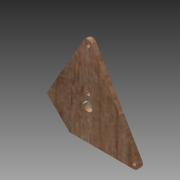
# Autodesk Inventor part: endPlateNew
Saved by Autodesk Inventor 2015 (Build 190159000, 159)
## iProperties
Created: 2014-11-20
Part Number: endPlateNew
Material: Wood (Birch)
Document SubType Name: Modeling
Designer: rawrdong
Density: 0.55 g/cm^3
Appearance: Birch - Natural Polished
Author: rawrdong
Autodesk Inventor part; units mm, degrees
ref_plane "YZ Plane" through (0, 0, 0) normal (1, 0, 0) x (0, 1, 0)
ref_plane "XZ Plane" through (0, 0, 0) normal (0, 1, 0) x (-1, 0, 0)
ref_plane "XY Plane" through (0, 0, 0) normal (0, 0, 1) x (1, 0, 0)
sketch "Sketch1" plane through (0, 0, 0) normal (0, 0, 1) x (1, 0, 0)
  arc A0 (24.3433, 15.7866) -> (20.9282, 16.7017) centre (22.1782, 14.5366) ccw projected
  line L0 (24.3433, 15.7866) -> (25.8433, 13.1886) projected
  arc A1 (24.9282, 9.7735) -> (25.8433, 13.1886) centre (23.6782, 11.9386) ccw projected
  line L1 (22.7631, 8.5235) -> (24.9282, 9.7735) projected
  arc A2 (22.7631, 8.5235) -> (22.0311, 5.7915) centre (23.7631, 6.7915) ccw projected
  line L2 (22.0311, 5.7915) -> (35.0311, -16.7252) projected
  arc A3 (32, -21.9752) -> (35.0311, -16.7252) centre (32, -18.4752) ccw projected
  line L3 (32, -21.9752) -> (6, -21.9752) projected
  arc A4 (6, -21.9752) -> (4, -23.9752) centre (6, -23.9752) ccw projected
  line L4 (4, -26.4752) -> (4, -23.9752) projected
  arc A5 (1.5, -28.9752) -> (4, -26.4752) centre (1.5, -26.4752) ccw projected
  line L5 (1.5, -28.9752) -> (-1.5, -28.9752) projected
  arc A6 (-4, -26.4752) -> (-1.5, -28.9752) centre (-1.5, -26.4752) ccw projected
  line L6 (-4, -23.9752) -> (-4, -26.4752) projected
  arc A7 (-4, -23.9752) -> (-6, -21.9752) centre (-6, -23.9752) ccw projected
  line L7 (-6, -21.9752) -> (-32, -21.9752) projected
  arc A8 (-35.0311, -16.7252) -> (-32, -21.9752) centre (-32, -18.4752) ccw projected
  line L8 (-35.0311, -16.7252) -> (-22.0311, 5.7915) projected
  arc A9 (-22.0311, 5.7915) -> (-22.7631, 8.5235) centre (-23.7631, 6.7915) ccw projected
  line L9 (-24.9282, 9.7735) -> (-22.7631, 8.5235) projected
  arc A10 (-25.8433, 13.1886) -> (-24.9282, 9.7735) centre (-23.6782, 11.9386) ccw projected
  line L10 (-25.8433, 13.1886) -> (-24.3433, 15.7866) projected
  arc A11 (-20.9282, 16.7017) -> (-24.3433, 15.7866) centre (-22.1782, 14.5366) ccw projected
  line L11 (-18.7631, 15.4517) -> (-20.9282, 16.7017) projected
  arc A12 (-18.7631, 15.4517) -> (-16.0311, 16.1838) centre (-17.7631, 17.1838) ccw projected
  line L12 (-16.0311, 16.1838) -> (-3.0311, 38.7004) projected
  arc A13 (3.0311, 38.7004) -> (-3.0311, 38.7004) centre (0, 36.9504) ccw projected
  line L13 (3.0311, 38.7004) -> (16.0311, 16.1838) projected
  arc A14 (16.0311, 16.1838) -> (18.7631, 15.4517) centre (17.7631, 17.1838) ccw projected
  line L14 (20.9282, 16.7017) -> (18.7631, 15.4517) projected
  circle A15 centre (22.6033, 13.05) radius 1.25 projected
  circle A16 centre (-22.6033, 13.05) radius 1.25 projected
  circle A17 centre (0, -26.1) radius 1.25 projected
  arc A18 (30.8494, -15.1698) -> (28.5621, -19.1315) centre (32, -18.4752) ccw projected
  arc A19 (30.8494, -15.1698) -> (31.118, -14.4475) centre (30.685, -14.6975) ccw projected
  line L15 (31.118, -14.4475) -> (3.0471, 34.1728) projected
  arc A20 (3.0471, 34.1728) -> (2.2873, 34.3012) centre (2.614, 33.9228) ccw projected
  arc A21 (-2.2873, 34.3012) -> (2.2873, 34.3012) centre (0, 36.9504) ccw projected
  arc A22 (-2.2873, 34.3012) -> (-3.0471, 34.1728) centre (-2.614, 33.9228) ccw projected
  line L16 (-3.0471, 34.1728) -> (-31.118, -14.4475) projected
  arc A23 (-31.118, -14.4475) -> (-30.8494, -15.1698) centre (-30.685, -14.6975) ccw projected
  arc A24 (-28.5621, -19.1315) -> (-30.8494, -15.1698) centre (-32, -18.4752) ccw projected
  arc A25 (-28.5621, -19.1315) -> (-28.0709, -19.7252) centre (-28.0709, -19.2252) ccw projected
  line L17 (-28.0709, -19.7252) -> (28.0709, -19.7252) projected
  arc A26 (28.0709, -19.7252) -> (28.5621, -19.1315) centre (28.0709, -19.2252) ccw projected
  circle A27 centre (-32, -18.4752) radius 1.4 projected
  circle A28 centre (0, 36.9504) radius 1.4 projected
  circle A29 centre (32, -18.4752) radius 1.4 projected
  line L18 (-15.7321, 16.7017) -> (-22.0311, 5.7915)
  line L19 (-6, -21.9752) -> (6, -21.9752)
  line L20 (22.0311, 5.7915) -> (16.0311, 16.1838)
  circle A30 centre (0, 0) radius 3.175
  circle A31 centre (0, 7.9) radius 1.425
  dimension "d2" = 6.35
  dimension "d3" = 2.85
  dimension "d4" = 7.9
  constraints: 6 end point, 2 centre point, 2 tangent, 1 coincident, 1 collinear, 1 horizontal, 1 point on line, 1 vertical alignment
  measures "d2" diameter of A30
  measures "d3" diameter of A31
  measures "d4" distance of point (0, 0) A31.centre
extrude "Extrusion1" add sketch "Sketch1" along normal blind 2.85 contours L20 L2 A3 L3 L19 L7 A8 L8 L18 L12 A13 L13 | A18 A26 L17 A25 A24 A23 L16 A22 A21 A20 L15 A19
body "Solid1"
